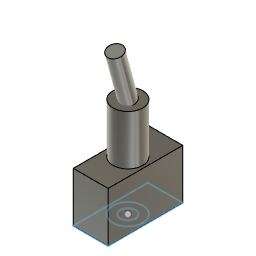
useless_box (Autodesk Fusion 360 archive; units mm, degrees)
design "small_switch"
Autodesk Fusion 360 part; units mm, degrees
note: some values were not read from the file. Chosen so that the rebuilt part matches the saved one: which bodies a step acts on; which face or edge a step refers to. Set by a fixed rule: which sketch regions a step uses.
sketch "Sketch1" plane through (0, 0, 0) normal (0, 0, 1) x (1, 0, 0)
  circle A0 centre (0, 0) radius 1.5
  circle A1 centre (0, 0) radius 3
  line L0 (3.5227, -7.5) -> (-3.4773, -7.5)
  line L1 (-3.4773, -7.5) -> (-3.4773, 7.5)
  line L2 (3.5227, 7.5) -> (3.5227, -7.5)
  line L3 (-3.4773, 7.5) -> (3.5227, 7.5)
  dimension "d20" = 6
  dimension "d29" = 3
  constraint horizontal L3
  constraint vertical L2
  constraint horizontal L0
  constraint vertical L1
  constraint concentric A0 A1
  measures "d20" diameter of A1
  measures "d29" diameter of A0
extrude "Extrude1" add sketch "Sketch1" along normal blind 30 and the other way blind -20 contours A0 makes body 1
extrude "Extrude2" add sketch "Sketch1" along normal blind 20 separate body contours A0 | A1 makes body 2
extrude "Extrude3" add sketch "Sketch1" along normal blind 10 separate body contours L0 L1 L2 L3 makes body 3
move_body "Move1" bodies 1 to x (1, 0, 0) y (0, 0.965926, 0.258819) z (0, -0.258819, 0.965926) at (0, 5.1764, 0.6815)

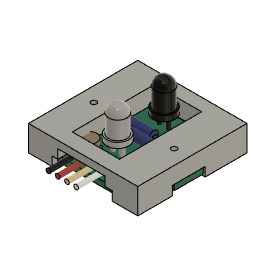
design "sensor"
Autodesk Fusion 360 part; units mm, degrees
sketch "Sketch1" plane through (0, 0, 0) normal (0, 0, 1) x (1, 0, 0)
  line L0 (0, 0) -> (15.24, 0)
  line L1 (15.24, 0) -> (15.24, 25.4)
  line L2 (15.24, 25.4) -> (0, 25.4)
  line L3 (0, 25.4) -> (0, 0)
  line L4 (2.54, 1.27) -> (12.7, 1.27)
  line L5 (12.7, 1.27) -> (12.7, 3.81)
  line L6 (12.7, 3.81) -> (2.54, 3.81)
  line L7 (2.54, 3.81) -> (2.54, 1.27)
  circle A0 centre (3.8195, 2.54) radius 0.635
  circle A1 centre (6.3595, 2.54) radius 0.635
  circle A2 centre (8.8995, 2.54) radius 0.635
  circle A3 centre (11.4395, 2.54) radius 0.635
  circle A4 centre (7.62, 8.89) radius 2.5
  line L8 (16.51, 21.59) -> (-7.62, 21.59) construction
  circle A5 centre (7.62, 21.59) radius 2.5
  line L9 (3.322, 17.78) -> (9.4206, 17.78)
  line L10 (9.4206, 17.78) -> (9.4206, 15.2896)
  line L11 (9.4206, 15.2896) -> (3.322, 15.2896)
  line L12 (3.322, 15.2896) -> (3.322, 17.78)
  circle A6 centre (6.35, 21.59) radius 0.635
  circle A7 centre (8.89, 21.59) radius 0.635
  circle A8 centre (6.35, 8.89) radius 0.635
  circle A9 centre (8.89, 8.89) radius 0.635
  circle A10 centre (6.35, 8.89) radius 0.635
  line L13 (11.8862, 12.7) -> (5.8127, 12.7)
  line L14 (5.8127, 12.7) -> (5.8127, 15.1867)
  line L15 (5.8127, 15.1867) -> (11.8862, 15.1867)
  line L16 (11.8862, 15.1867) -> (11.8862, 12.7)
  circle A11 centre (2.54, 16.51) radius 0.635
  circle A12 centre (10.16, 16.51) radius 0.635
  circle A13 centre (5.08, 13.97) radius 0.635
  circle A14 centre (12.7, 13.97) radius 0.635
  circle A15 centre (7.62, 8.89) radius 3
  circle A16 centre (7.62, 21.59) radius 3
  circle A17 centre (3.8195, 5.08) radius 0.635
  circle A18 centre (3.8195, 7.62) radius 0.635
  circle A19 centre (2.2166, 6.3624) radius 2.1559
  line L17 (-7, 17) -> (-7, 9)
  line L18 (-7, 17) -> (0, 17)
  line L19 (-7, 9) -> (0, 9)
  line L20 (15.24, 17) -> (23, 17)
  line L21 (23, 17) -> (23, 10)
  line L22 (23, 10) -> (23, 9)
  line L23 (23, 9) -> (15.24, 9)
  circle A20 centre (-3, 12.9629) radius 1.25
  circle A21 centre (19, 13) radius 1.25
  dimension "d1" = 15.24
  dimension "d2" = 25.4
  dimension "d3" = 1.27
  dimension "d6" = 7.62
  dimension "d7" = 0
  dimension "d8" = 5
  dimension "d9" = 5
  dimension "d10" = 1.27
  dimension "d11" = 1.27
  dimension "d12" = 1.27
  dimension "d13" = 1.27
  dimension "d14" = 1.27
  dimension "d15" = 1.27
  dimension "d16" = 1.27
  dimension "d17" = 1.27
  dimension "d18" = 1.27
  dimension "d19" = 6
  dimension "d20" = 6
  dimension "d43" = 1.27
  dimension "d44" = 1.27
  dimension "d53" = 2.5
  dimension "d54" = 2.5
  dimension "d55" = 22
  constraint horizontal L0
  constraint vertical L1
  constraint horizontal L2
  constraint vertical L3
  constraint coincident L0.start L3.end
  constraint horizontal L4
  constraint vertical L5
  constraint horizontal L6
  constraint vertical L7
  constraint perpendicular L1 L8
  constraint coincident L8 A5.centre
  constraint horizontal L9
  constraint vertical L10
  constraint horizontal L11
  constraint vertical L12
  constraint coincident L8 A6.centre
  constraint horizontal L13
  constraint vertical L14
  constraint horizontal L15
  constraint vertical L16
  constraint concentric A4 A15
  constraint concentric A5 A16
  constraint perpendicular L8 L17
  constraint coincident L3 L18.end
  constraint perpendicular L3 L18
  constraint coincident L3 L19.end
  constraint perpendicular L3 L19
  constraint coincident L1 L20.start
  constraint perpendicular L1 L20
  constraint perpendicular L20 L21
  constraint perpendicular L20 L22
  constraint coincident L1 L23.end
  constraint perpendicular L1 L23
  measures "d1" distance of L0.start L0.end
  measures "d2" distance of L0.start L2.end
  measures "d3" diameter of A0
  measures "d8" diameter of A4
  measures "d9" diameter of A5
  measures "d10" diameter of A6
  measures "d11" diameter of A7
  measures "d12" diameter of A8
  measures "d13" diameter of A9
  measures "d14" diameter of A10
  measures "d15" diameter of A11
  measures "d16" diameter of A12
  measures "d17" diameter of A13
  measures "d18" diameter of A14
  measures "d19" diameter of A15
  measures "d20" diameter of A16
  measures "d43" diameter of A17
  measures "d44" diameter of A18
  measures "d53" diameter of A20
  measures "d54" diameter of A21
  measures "d55" horizontal distance of A20.centre A21.centre
sketch "Sketch2" plane through (0, 0, 0) normal (1, 0, 0) x (0, 1, 0)
  arc A0 through (2.54, 0, 3.81) (2.168, 0.898, 3.81) (1.27, 1.27, 3.81)
  line L0 (-6.35, 1.27, 3.81) -> (1.27, 1.27, 3.81)
  arc A1 through (2.54, 0, 6.35) (2.168, 0.898, 6.35) (1.27, 1.27, 6.35)
  line L1 (-6.35, 1.27, 6.35) -> (1.27, 1.27, 6.35)
  arc A2 through (2.54, 0, 8.89) (2.168, 0.898, 8.89) (1.27, 1.27, 8.89)
  line L2 (-6.35, 1.27, 8.89) -> (1.27, 1.27, 8.89)
  arc A3 through (2.54, 0, 11.43) (2.168, 0.898, 11.43) (1.27, 1.27, 11.43)
  line L3 (-6.35, 1.27, 11.43) -> (1.27, 1.27, 11.43)
  circle A4 centre (16.51, 1.27) radius 1.25
  circle A5 centre (13.97, 1.27) radius 1.25
  dimension "d26" = 2.5
  dimension "d27" = 2.5
  measures "d26" diameter of A4
  measures "d27" diameter of A5
extrude "Extrude1" add sketch "Sketch1" along normal blind 6.5 contours A4 | A5 | A6 | A7 | A8 A10 | A9 makes body 1 at (10.1076, 21.3411, 4.3333) makes body 2 at (10.1076, 8.6411, 4.3333)
sphere "SpherePrimitive1" add diameter 5 placed x (-1, 0, 0) y (0, -1, 0) z (0, 0, 1) at (7.62, 21.59, 6.5) bodies 1
extrude "Extrude2" add sketch "Sketch1" along normal blind 1.5 contours A15 | A16 bodies 1 2
sphere "SpherePrimitive2" add diameter 5.0038 placed x (-1, 0, 0) y (0, -1, 0) z (0, 0, 1) at (7.62, 8.89, 6.5) bodies 2
sweep "Sweep1" add profiles "Sketch1" path "Sketch2" along L0 A0 section 1 contours A0 | A1 | A2 | A3 separate body makes body 3 at (6.9914, -1.27, 1.3332) makes body 4 at (9.5314, -1.27, 1.3332) makes body 5 at (4.4514, -1.27, 1.3332) makes body 6 at (12.0714, -1.27, 1.3332)
extrude "Extrude3" add sketch "Sketch2" along normal blind 9.906 and the other way blind -2.794 separate body contours A4 makes body 7
extrude "Extrude4" add sketch "Sketch2" along normal blind 12.446 and the other way blind -5.334 separate body contours A5 makes body 8
extrude "Extrude5" add sketch "Sketch1" along normal blind 2 separate body contours A17 A19 | A17 A18 A19 | A18 A19 picked at (3.5895, 4.9795) picked at (3.8746, 7.3788) makes body 9
extrude "Extrude6" add sketch "Sketch1" against normal blind 2.5 contours A0 | A1 | A2 | A3 | A6 | A7 | A8 A10 | A9 | A11 | A12 | A13 | A14 | A17 A19 | A17 A19 | A18 A19 | A18 A19 bodies 1 2 3 4 5 6 9 makes body 10 at (13.2418, 14.3011, -1.6667) makes body 11 at (4.5382, 13.6389, -1.6667) makes body 12 at (9.6736, 16.9182, -1.6667) makes body 13 at (1.9082, 16.4468, -1.6667)
extrude "Extrude7" add sketch "Sketch1" along normal blind 1.27 contours A11 | A12 | A13 | A14 bodies 7 8 10 11 12 13
extrude "Extrude8" add sketch "Sketch1" against normal blind 1.5 separate body contours L0 L1 L2 L3 | L3 L17 L18 L19 | L1 L20 L21 L22 L23 | L4 L5 L6 L7 | A0 | A1 | A2 | A3 | A4 | A5 | L9 L10 L11 L12 | A6 | A7 | A8 A10 | A9 | L13 L14 L15 L16 | A11 | A12 | A13 | A14 | A15 | A16 | A17 A19 | A17 A19 | A17 A18 A19 | A18 A19 | A18 A19 makes body 14
move_body "Move1" bodies 1 2 to x (1, 0, 0) y (0, 1, 0) z (0, 0, 1) at (0, 0, 3)
extrude "Extrude9" add 4 faces at (6.2674, 22.0322, 0.5) (9.0452, 21.8588, 0.5) (8.758, 8.5408, 0.5) (6.5249, 9.0092, 0.5) along direction (0, 0, -1) blind 3 on bodies 1 2 bodies 1 2
ref_plane "WorkPlane1" through (0, 0, 4.5) normal (0, 0, 1) x (1, 0, 0) in component "sensor_mount"
ref_plane "WorkPlane2" through (0, 0, 9.125) normal (0, 0, 1) x (1, 0, 0) in component "sensor_mount"
sketch "Sketch1 (2)" plane through (0, 0, 4.5) normal (0, 0, 1) x (1, 0, 0) in component "sensor_mount"
  line L0 (-7, 29) -> (23, 29)
  line L1 (23, 29) -> (23, -1)
  line L2 (23, -1) -> (-7, -1)
  line L3 (-7, -1) -> (-7, 29)
  line L4 (14, 32) -> (14, -1)
  line L5 (1.0449, -1) -> (1.0449, 29)
  line L6 (14, 25.5493) -> (1.0449, 25.5493)
  line L7 (14, 3) -> (1.0449, 3)
  circle A0 centre (19, 13) radius 0.75
  circle A1 centre (-3, 12.9629) radius 0.75
  line L8 (-0.5, 17.5) -> (-7, 17.5)
  line L9 (-0.5, 8.5) -> (-7, 8.5)
  line L10 (16, 8.5) -> (23, 8.5)
  line L11 (16, 17.5) -> (23, 17.5)
  line L12 (16, 17.5) -> (16, 29)
  line L13 (16, 8.5) -> (16, -1)
  line L14 (-0.5, 8.5) -> (-0.5, -1)
  line L15 (-0.5, 17.5) -> (-0.5, 29)
  point P0 (19, 13)
  point P1 (-3, 12.9629)
  dimension "d72" = 1.5
  dimension "d73" = 1.5
  constraint horizontal L0
  constraint vertical L1
  constraint horizontal L2
  constraint vertical L3
  constraint coincident L2 L4.end
  constraint perpendicular L2 L4
  constraint coincident L2 L5.start
  constraint coincident L0 L5.end
  constraint perpendicular L0 L5
  constraint coincident L4 L6.start
  constraint coincident L5 L6.end
  constraint perpendicular L5 L6
  constraint coincident L5 L7.end
  constraint perpendicular L5 L7
  constraint coincident P0 A0.centre
  constraint coincident P1 A1.centre
  constraint coincident L3 L8.end
  constraint perpendicular L3 L8
  constraint coincident L3 L9.end
  constraint perpendicular L3 L9
  constraint coincident L1 L10.end
  constraint perpendicular L1 L10
  constraint coincident L1 L11.end
  constraint perpendicular L1 L11
  constraint coincident L0 L12.end
  constraint perpendicular L0 L12
  constraint coincident L2 L13.end
  constraint perpendicular L2 L13
  constraint coincident L2 L14.end
  constraint perpendicular L2 L14
  constraint coincident L0 L15.end
  constraint perpendicular L0 L15
  measures "d72" diameter of A0
  measures "d73" diameter of A1
extrude "Extrude4'" add sketch "Sketch1 (2)" against normal blind 4.5 separate body contours L0 L3 L8 L15 | L0 L2 L3 L5 L8 L9 L14 L15 | L0 L4 L5 L6 | L2 L3 L9 L14 | L0 L1 L2 L4 L10 L11 L12 L13 | L0 L1 L11 L12 | L1 L2 L10 L13 makes body 15 in component "sensor_mount"
extrude "Extrude5'" add sketch "Sketch1 (2)" against normal blind 2 contours L2 L4 L5 L7 bodies 15 in component "sensor_mount"
extrude "Extrude6'" add sketch "Sketch1 (2)" against normal blind 7 contours L0 L3 L8 L15 | L2 L3 L9 L14 | L0 L1 L11 L12 | L1 L2 L10 L13 bodies 15 in component "sensor_mount"
component "sensor_mount" placed x (1, 0, 0) y (0, 1, 0) z (0, 0, 1) at (0, 0, 0)
named bodies: "detector", "emitter", "wire2", "wire3", "wire1", "wir45", "res1", "res2", "cap", "board"

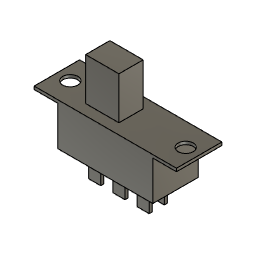
design "slide_switch"
Autodesk Fusion 360 part; units mm, degrees
sketch "Sketch1" plane through (0, 0, 0) normal (0, 0, 1) x (1, 0, 0)
  line L0 (11.75, 3.75) -> (-11.75, 3.75)
  line L1 (-11.75, 3.75) -> (-11.75, -3.75)
  line L2 (-11.75, -3.75) -> (11.75, -3.75)
  line L3 (11.75, -3.75) -> (11.75, 3.75)
  line L4 (11.75, 3.75) -> (-11.75, -3.75) construction
  line L5 (-11.75, 3.75) -> (11.75, -3.75) construction
  line L6 (7.85, -3.75) -> (-7.85, -3.75)
  line L7 (-7.85, -3.75) -> (-7.85, 3.75)
  line L8 (-7.85, 3.75) -> (7.85, 3.75)
  line L9 (7.85, 3.75) -> (7.85, -3.75)
  line L10 (7.85, -3.75) -> (-7.85, 3.75) construction
  line L11 (-7.85, -3.75) -> (7.85, 3.75) construction
  line L12 (9.525, -3.75) -> (-9.525, -3.75) construction
  line L13 (-9.525, -3.75) -> (-9.525, 3.75) construction
  line L14 (-9.525, 3.75) -> (9.525, 3.75) construction
  line L15 (9.525, 3.75) -> (9.525, -3.75) construction
  line L16 (9.525, -3.75) -> (-9.525, 3.75) construction
  line L17 (-9.525, -3.75) -> (9.525, 3.75) construction
  circle A0 centre (-9.525, 0) radius 1.25
  circle A1 centre (9.525, 0) radius 1.25
  line L18 (5, 2) -> (-5, 2) construction
  line L19 (-5, 2) -> (-5, -2) construction
  line L20 (-5, -2) -> (5, -2) construction
  line L21 (5, -2) -> (5, 2) construction
  line L22 (5, 2) -> (-5, -2) construction
  line L23 (-5, 2) -> (5, -2) construction
  line L24 (-5, 2) -> (0.5, 2)
  line L25 (0.5, 2) -> (0.5, -2)
  line L26 (0.5, -2) -> (-5, -2)
  line L27 (-5, -2) -> (-5, 2)
  dimension "d1" = 23.5
  dimension "d2" = 7.5
  dimension "d3" = 15.7
  dimension "d4" = 19.05
  dimension "d5" = 2.5
  dimension "d6" = 2.5
  dimension "d7" = 10
  dimension "d8" = 4
  dimension "d9" = 5.5
  constraint horizontal L0
  constraint perpendicular L0 L1
  constraint parallel L0 L2
  constraint parallel L1 L3
  constraint coincident L4 origin
  constraint coincident L5 origin
  constraint horizontal L6
  constraint perpendicular L6 L7
  constraint parallel L6 L8
  constraint parallel L7 L9
  constraint coincident L10 origin
  constraint coincident L11 origin
  constraint coincident L2 L6.start
  constraint horizontal L12
  constraint perpendicular L12 L13
  constraint parallel L12 L14
  constraint parallel L13 L15
  constraint coincident L16 origin
  constraint coincident L17 origin
  constraint midpoint L13 A0.centre
  constraint midpoint L15 A1.centre
  constraint horizontal L18
  constraint perpendicular L18 L19
  constraint parallel L18 L20
  constraint parallel L19 L21
  constraint coincident L22 origin
  constraint coincident L23 origin
  constraint horizontal L24
  constraint vertical L25
  constraint horizontal L26
  constraint vertical L27
  measures "d1" distance of L1.end L2.end
  measures "d2" distance of L0.end L1.end
  measures "d3" distance of L7.end L8.end
  measures "d4" distance of L13.end L14.end
  measures "d5" diameter of A0
  measures "d6" diameter of A1
  measures "d7" distance of L19.end L20.end
  measures "d8" distance of L18.end L19.end
  measures "d9" distance of L18.end L24.end
extrude "Extrude1" add sketch "Sketch1" against normal blind 7 contours L0 L2 L6 L7 L8 L9 | L24 L25 L26 L27 makes body 1
extrude "Extrude2" add sketch "Sketch1" against normal blind 0.5 contours L0 L2 L3 L9 | L0 L1 L2 L7 bodies 1
extrude "Extrude3" add sketch "Sketch1" along normal blind 7 separate body contours L24 L25 L26 L27 makes body 2
sketch "Sketch2" plane through (0, 0, -7) normal (0, 0, -1) x (1, 0, 0)
  line L0 (-7.85, -3.75) -> (7.85, -3.75)
  line L1 (7.85, -3.75) -> (7.85, 3.75)
  line L2 (7.85, 3.75) -> (-7.85, 3.75)
  line L3 (-7.85, 3.75) -> (-7.85, -3.75)
  line L4 (-5, 1.5) -> (5, 1.5) construction
  line L5 (5, 1.5) -> (5, -1.5) construction
  line L6 (5, -1.5) -> (-5, -1.5) construction
  line L7 (-5, -1.5) -> (-5, 1.5) construction
  line L8 (-5, 1.5) -> (5, -1.5) construction
  line L9 (5, 1.5) -> (-5, -1.5) construction
  line L10 (-5, 1.5) -> (-3, 1.5)
  line L11 (-3, 1.5) -> (-3, 1)
  line L12 (-3, 1) -> (-5, 1)
  line L13 (-5, 1) -> (-5, 1.5)
  line L14 (-5, -1) -> (-3, -1)
  line L15 (-3, -1) -> (-3, -1.5)
  line L16 (-3, -1.5) -> (-5, -1.5)
  line L17 (-5, -1.5) -> (-5, -1)
  line L18 (-5, 1) -> (-5, 1.5)
  line L19 (-5, 1.5) -> (-3, 1.5)
  line L20 (-3, 1.5) -> (-3, 1)
  line L21 (-3, 1) -> (-5, 1)
  line L22 (5, 1.5) -> (-5, -1.5) construction
  line L23 (3, 1.5) -> (5, 1.5)
  line L24 (5, 1.5) -> (5, 1)
  line L25 (5, 1) -> (3, 1)
  line L26 (3, 1) -> (3, 1.5)
  line L27 (5, -1.5) -> (3, -1.5)
  line L28 (3, -1.5) -> (3, -1)
  line L29 (5, -1) -> (5, -1.5)
  line L30 (3, -1) -> (5, -1)
  line L31 (-1, 1.5) -> (1, 1.5)
  line L32 (1, 1.5) -> (1, 1)
  line L33 (1, 1) -> (-1, 1)
  line L34 (-1, 1) -> (-1, 1.5)
  line L35 (1, -1.5) -> (-1, -1.5)
  line L36 (-1, -1.5) -> (-1, -1)
  line L37 (1, -1) -> (1, -1.5)
  line L38 (-1, -1) -> (1, -1)
  dimension "d16" = 10
  dimension "d17" = 3
  dimension "d18" = 2
  dimension "d19" = 0.5
  dimension "d20" = 2
  dimension "d21" = 0.5
  dimension "d22" = 2
  dimension "d23" = 0.5
  dimension "d24" = 2
  dimension "d25" = 0.5
  dimension "d26" = 2
  dimension "d27" = 0.5
  dimension "d28" = 2
  dimension "d29" = 0.5
  dimension "d30" = 2
  dimension "d31" = 0.5
  constraint horizontal L4
  constraint perpendicular L4 L5
  constraint parallel L4 L6
  constraint parallel L5 L7
  constraint coincident L8 origin
  constraint coincident L9 origin
  constraint horizontal L10
  constraint vertical L11
  constraint horizontal L12
  constraint vertical L13
  constraint horizontal L14
  constraint vertical L15
  constraint horizontal L16
  constraint vertical L17
  constraint horizontal L19
  constraint vertical L20
  constraint horizontal L21
  constraint vertical L18
  constraint horizontal L23
  constraint vertical L24
  constraint horizontal L25
  constraint vertical L26
  constraint horizontal L30
  constraint vertical L29
  constraint horizontal L27
  constraint vertical L28
  constraint horizontal L31
  constraint vertical L32
  constraint horizontal L33
  constraint vertical L34
  constraint horizontal L38
  constraint vertical L37
  constraint horizontal L35
  constraint vertical L36
  measures "d16" distance of L5.end L6.end
  measures "d17" distance of L4.end L5.end
  measures "d18" distance of L4.start L10.end
  measures "d19" distance of L4.start L12.end
  measures "d20" distance of L14.end L14.start
  measures "d21" distance of L6.end L14.start
  measures "d22" distance of L10.end L4.start
  measures "d23" distance of L12.end L4.start
  measures "d24" distance of L4.end L23.start
  measures "d25" distance of L25.end L23.start
  measures "d26" distance of L28.end L29.start
  measures "d27" distance of L27.end L28.end
  measures "d28" distance of L31.end L31.start
  measures "d29" distance of L33.end L31.start
  measures "d30" distance of L36.end L37.start
  measures "d31" distance of L35.end L36.end
extrude "Extrude4" add sketch "Sketch2" along normal blind 4 contours L10 L11 L12 L13 L18 L19 L20 L21 | L14 L15 L16 L17 | L23 L24 L25 L26 | L27 L28 L29 L30 | L31 L32 L33 L34 | L35 L36 L37 L38 bodies 1 2
copy_body "Body->Comp1" bodies 1 removing the originals makes body 4 in component "body"
copy_body "Body->Comp2" bodies 2 removing the originals makes body 5 in component "slider"
component "body" placed x (1, 0, 0) y (0, 1, 0) z (0, 0, 1) at (0, 0, 0)
component "slider" placed x (1, 0, 0) y (0, 1, 0) z (0, 0, 1) at (0, 0, 0)
named bodies: "body", "slider"

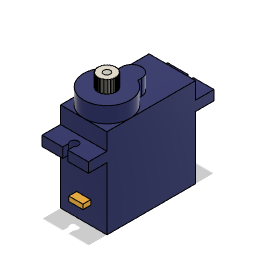
design "blue_SG90"
Autodesk Fusion 360 part; units mm, degrees
sketch "Left" plane through (0, 0, 0) normal (1, 0, 0) x (0, 0, -1)
  line L0 (-21.4055, -22.0984) -> (1.0945, -22.0984)
  line L1 (-21.4055, 4.6016) -> (1.0945, 4.6016)
  line L2 (-21.4055, 0.6016) -> (1.0945, 0.6016)
  line L3 (-21.4055, 0.6016) -> (-21.4055, 4.6016)
  line L4 (5.7945, -22.0984) -> (5.7945, -6.1984)
  line L5 (-26.1055, -6.1984) -> (-26.1055, -3.6984)
  line L6 (-26.1055, -3.6984) -> (-21.4055, -3.6984)
  line L7 (1.0945, -3.6984) -> (5.7945, -3.6984)
  line L8 (-26.1055, -6.1984) -> (-21.4055, -6.1984)
  line L9 (1.0945, -6.1984) -> (5.7945, -6.1984)
  line L10 (1.0945, -22.0984) -> (1.0945, -6.1984)
  line L11 (1.0945, -3.6984) -> (1.0945, 0.6016)
  line L12 (-21.4055, -22.0984) -> (-21.4055, -6.1984)
  line L13 (-21.4055, -3.6984) -> (-21.4055, 0.6016)
  line L14 (-15.5055, 0.6016) -> (-15.5055, 13)
  line L15 (-6.7055, 0.6016) -> (-6.7055, 13)
  line L16 (1.0945, -22.0984) -> (1.0945, -6.1984)
  line L17 (1.0945, -3.6984) -> (1.0945, 13)
  line L18 (5.7945, -3.6984) -> (5.7945, -6.1984)
  dimension "d1" = 22.5
  dimension "d2" = 26.7
  dimension "d3" = 22.7
  dimension "d4" = 4
  dimension "d5" = 22.7
  dimension "d13" = 5.9
  constraint perpendicular L1 L3
  constraint parallel L0 L6
  constraint parallel L0 L8
  constraint parallel L5 L12
  constraint coincident L6.end L12
  constraint coincident L7.start L10
  constraint collinear L6 L7
  constraint collinear L8 L9
  constraint parallel L4 L10
  constraint collinear L10 L11
  constraint collinear L12 L13
  constraint parallel L3 L14
  constraint parallel L14 L16
  constraint collinear L16 L17
  constraint parallel L14 L15
  constraint coincident L2 L15.start
  constraint coincident L2 L14.start
  constraint perpendicular L9 L18
  measures "d1" distance of L0.start L0.end
  measures "d4" distance of L1.start L2.start
  measures "d5" distance of L0.start L2.start
  measures "d13" distance of L3 L14
extrude "Extrude1" add sketch "Left" along normal mid plane 11.8 contours L0 L2 L5 L6 L7 L8 L9 L10 L11 L12 L13 L16 L17 L18 makes body 1
sketch "TOP" plane through (0, 0.6016, 0) normal (0, 1, 0) x (-1, 0, 0)
  line L0 (5.9, 21.4055) -> (-5.9, 21.4055)
  line L1 (-5.9, 21.4055) -> (-5.9, -1.0945)
  line L2 (-5.9, -1.0945) -> (5.9, -1.0945)
  line L3 (5.9, -1.0945) -> (5.9, 21.4055)
  circle A0 centre (0, 15.5055) radius 2.3
  circle A1 centre (0, 15.5055) radius 0.85
  line L4 (0, -1.0945) -> (0, 27)
  line L5 (0, 27) -> (0, -1.0945)
  arc A2 (-2.5, 9.2055) -> (2.5, 9.2055) centre (0, 9.2055) ccw
  line L6 (-2.5, 9.2055) -> (-2.5, 10.1613)
  line L7 (2.5, 9.2055) -> (2.5, 10.1613)
  arc A3 (2.5, 10.1613) -> (-2.5, 10.1613) centre (0, 15.5055) ccw
  line L8 (5.9, -5.7945) -> (-5.9, -5.7945)
  line L9 (-0.65, -4.2545) -> (-0.65, -5.7945)
  line L10 (0.65, -4.2545) -> (0.65, -5.7945)
  arc A4 (0.65, -4.2545) -> (-0.65, -4.2545) centre (0, -3.4945) ccw
  line L11 (5.9, 26.1055) -> (-5.9, 26.1055)
  arc A5 (-0.65, 24.5654) -> (0.65, 24.5654) centre (0, 23.8055) ccw
  line L12 (0.65, 24.5654) -> (0.65, 26.1055)
  line L13 (-0.65, 24.5654) -> (-0.65, 26.1055)
  point P0 (0, 15.5055)
  point P1 (0, 6.7055)
  point P2 (0, -1.0945)
  point P3 (5.9, -5.7945)
  point P4 (-5.9, -5.7945)
  point P5 (0, -5.7945)
  point P6 (5.9, 26.1055)
  point P7 (-5.9, 26.1055)
  point P8 (0, 26.1055)
  point P9 (0, 21.4055)
  dimension "d16" = 4.6
  dimension "d17" = 1.7
  dimension "d18" = 11.8
  dimension "d27" = 2
  dimension "d31" = 2
  constraint coincident P0 A0.centre
  constraint concentric A1 A3
  constraint coincident P1 A2
  constraint coincident P2 L4.start
  constraint perpendicular L0 L4
  constraint parallel L4 L6
  constraint parallel L4 L7
  constraint coincident P3 L8.start
  constraint coincident P4 L8.end
  constraint coincident P6 L11.start
  constraint coincident P7 L11.end
  constraint coincident L11 L12.end
  constraint coincident L11 L13.end
  measures "d16" diameter of A0
  measures "d17" diameter of A1
  measures "d18" diameter of A3
  measures "d27" diameter of A4
  measures "d31" diameter of A5
extrude "Extrude2" add sketch "TOP" along normal blind 4 contours A0 L4 L5 A2 L7 A3 | A0 L4 L5 A2 L6 A3 bodies 1
extrude "Extrude3" add sketch "TOP" along normal blind 7.2 separate body contours A0 A1 L4 L5 | A0 A1 L4 L5 makes body 2
extrude "Extrude4" cut sketch "TOP" against normal through all contours L4 L5 L11 A5 L13 | L4 L5 L11 A5 L12 bodies 1
extrude "Extrude5" cut sketch "TOP" against normal through all contours L8 L9 L10 A4 bodies 1
sketch "Front" plane through (0, 0, 21.4055) normal (0, 0, 1) x (1, 0, 0)
  line L0 (-5.9, -22.0984) -> (5.9, -22.0984)
  line L1 (5.9, -22.0984) -> (5.9, -6.1984)
  line L2 (5.9, -6.1984) -> (-5.9, -6.1984)
  line L3 (-5.9, -6.1984) -> (-5.9, -22.0984)
  line L4 (-1.8, -17.5984) -> (1.8, -17.5984)
  line L5 (0, -22.0984) -> (0, -6.1984)
  line L6 (1.8, -17.5984) -> (1.8, -16.3984)
  line L7 (-1.8, -17.5984) -> (-1.8, -16.3984)
  line L8 (-1.8, -16.3984) -> (1.8, -16.3984)
extrude "Extrude6" add sketch "Front" along normal blind 2 separate body contours L4 L5 L6 L8 | L4 L5 L7 L8 makes body 3
copy_body "Body->Comp1" bodies 3 removing the originals makes body 4 in component "connector"
copy_body "Body->Comp2" bodies 2 removing the originals makes body 5 in component "shaft"
copy_body "Body->Comp3" bodies 1 removing the originals makes body 6 in component "body\\"
sketch "Sketch1" plane through (0, 7.8016, 0) normal (0, 1, 0) x (-1, 0, 0) in component "shaft"
  circle A0 centre (0, 15.5055) radius 0.85
  circle A1 centre (0, 15.5055) radius 2.3
  circle A2 centre (0, 15.5055) radius 2.3
  circle A3 centre (-0.0134, 13.2055) radius 0.125
  dimension "d42" = 0.25
  constraint coincident A2 A3.centre
  measures "d42" diameter of A3
extrude "Extrude1'" cut sketch "Sketch1" against normal up to surface (3.2 mm away) contours A1 A2 A3 | A1 A2 A3 picked at (-0.0101, 13.2473) picked at (-0.0141, 13.1641) bodies 5 in component "shaft"
pattern_circular "C-Pattern1" count 28 over 360 about axis through (0, 15.4797, 15.5055) along (0, -1, 0) of "Extrude1'" in component "shaft"
component "connector" placed x (1, 0, 0) y (0, 1, 0) z (0, 0, 1) at (0, 0, 0)
component "shaft" placed x (1, 0, 0) y (0, 1, 0) z (0, 0, 1) at (0, 0, 0)
component "body\\" placed x (1, 0, 0) y (0, 1, 0) z (0, 0, 1) at (0, 0, 0)

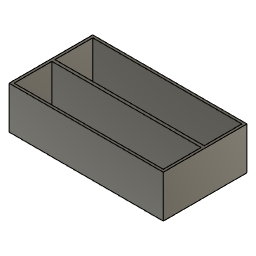
design "battery_holder"
Autodesk Fusion 360 part; units mm, degrees
sketch "Sketch1" plane through (0, 0, 0) normal (0, 0, 1) x (1, 0, 0)
  line L0 (38.25, 20.75) -> (-38.25, 20.75)
  line L1 (-38.25, 20.75) -> (-38.25, -20.75)
  line L2 (-38.25, -20.75) -> (38.25, -20.75)
  line L3 (38.25, -20.75) -> (38.25, 20.75)
  line L4 (38.25, 20.75) -> (-38.25, -20.75) construction
  line L5 (-38.25, 20.75) -> (38.25, -20.75) construction
  line L6 (-37, 19.5) -> (37, 19.5)
  line L7 (37, 19.5) -> (37, -19.5)
  line L8 (37, -19.5) -> (-37, -19.5)
  line L9 (-37, -19.5) -> (-37, 19.5)
  line L10 (-37, 19.5) -> (37, -19.5) construction
  line L11 (37, 19.5) -> (-37, -19.5) construction
  line L12 (37, -0.75) -> (-37, -0.75)
  line L13 (-37, -0.75) -> (-37, 0.75)
  line L14 (-37, 0.75) -> (37, 0.75)
  line L15 (37, 0.75) -> (37, -0.75)
  line L16 (37, -0.75) -> (-37, 0.75) construction
  line L17 (-37, -0.75) -> (37, 0.75) construction
  line L18 (0, 0) -> (0, 10) construction
  line L19 (0, 0) -> (0, -10) construction
  circle A0 centre (0, -10) radius 1.5
  circle A1 centre (0, 10) radius 1.5
  dimension "d1" = 76.5
  dimension "d2" = 41.5
  dimension "d3" = 74
  dimension "d4" = 39
  dimension "d5" = 1.5
  dimension "d10" = 10
  dimension "d11" = 10
  dimension "d12" = 3
  dimension "d13" = 3
  constraint horizontal L0
  constraint perpendicular L0 L1
  constraint parallel L0 L2
  constraint parallel L1 L3
  constraint coincident L4 L18.start
  constraint coincident L5 L18.start
  constraint coincident L18.start L19.start
  constraint horizontal L6
  constraint perpendicular L6 L7
  constraint parallel L6 L8
  constraint parallel L7 L9
  constraint coincident L10 L18.start
  constraint coincident L11 L18.start
  constraint horizontal L12
  constraint perpendicular L12 L13
  constraint parallel L12 L14
  constraint parallel L13 L15
  constraint coincident L16 L18.start
  constraint coincident L17 L18.start
  constraint vertical L18
  constraint vertical L19
  constraint coincident L19.end A0.centre
  constraint coincident L18.end A1.centre
  measures "d1" distance of L1.end L2.end
  measures "d2" distance of L0.end L1.end
  measures "d3" distance of L7.end L8.end
  measures "d4" distance of L6.end L7.end
  measures "d5" distance of L12.end L13.end
  measures "d10" distance of L18.start L18.end
  measures "d11" distance of L18.start L19.end
  measures "d12" diameter of A0
  measures "d13" diameter of A1
extrude "Extrude1" add sketch "Sketch1" along normal blind 21 contours L0 L1 L2 L3 | L7 L9 L12 L13 L14 L15
extrude "Extrude2" add sketch "Sketch1" along normal blind 1.5 contours L6 L7 L9 L14 | L7 L8 L9 L12

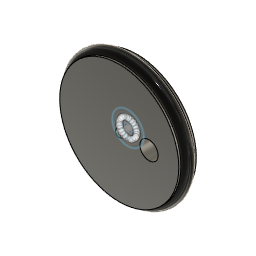
design "wheel"
Autodesk Fusion 360 part; units mm, degrees
sketch "servo splines" plane through (0, 0, 0) normal (0, 1, 0) x (1, 0, 0)
  circle A0 centre (0, 0) radius 1.1
  circle A1 centre (0, 0) radius 4.5
  circle A2 centre (0, 0) radius 2.2
  line L0 (-0.9545, -1.9821) -> (-0.822, -2.361)
  line L1 (1.72, 1.3717) -> (2.1189, 1.3267)
  line L2 (0.9545, -1.9821) -> (0.822, -2.361)
  line L3 (2.1448, -0.4895) -> (2.3584, -0.8294)
  line L4 (-1.9053, -1.1) -> (-2.293, -0.9961)
  line L5 (-2.1448, -0.4895) -> (-2.4847, -0.276)
  line L6 (-1.4964, -1.6127) -> (-1.4814, -2.0138)
  line L7 (-0.3279, -2.1754) -> (-0.6509, -2.4138)
  line L8 (-2.0479, 0.8038) -> (-2.2084, 1.1717)
  line L9 (-1.2393, 1.8177) -> (-1.6337, 1.8924)
  line L10 (0.9545, -1.9821) -> (1.3334, -2.1147)
  line L11 (2.1938, 0.1644) -> (2.4557, 0.4687)
  line L12 (-1.9053, -1.1) -> (-2.0091, -1.4877)
  line L13 (1.9053, -1.1) -> (2.0091, -1.4877)
  line L14 (0.3279, -2.1754) -> (0.0895, -2.4984)
  line L15 (1.2393, 1.8177) -> (1.6337, 1.8924)
  line L16 (0.6485, 2.1023) -> (0.4609, 2.4571)
  line L17 (-2.1938, 0.1644) -> (-2.4981, -0.0974)
  line L18 (0, 2.2) -> (-0.2838, 2.4838)
  line L19 (-1.4964, -1.6127) -> (-1.8975, -1.6277)
  line L20 (-1.2393, 1.8177) -> (-1.1647, 2.2121)
  line L21 (-1.72, 1.3717) -> (-2.1189, 1.3267)
  line L22 (0, 2.2) -> (0.2838, 2.4838)
  line L23 (1.2393, 1.8177) -> (1.1647, 2.2121)
  line L24 (-1.72, 1.3717) -> (-1.765, 1.7706)
  line L25 (-0.6485, 2.1023) -> (-1.0033, 2.2898)
  line L26 (2.1448, -0.4895) -> (2.4847, -0.276)
  line L27 (0, 0) -> (0, 4.5) construction
  circle A3 centre (0, 0) radius 2.5
  line L28 (-0.3279, -2.1754) -> (-0.0895, -2.4984)
  line L29 (2.0479, 0.8038) -> (2.2084, 1.1717)
  line L30 (2.0479, 0.8038) -> (2.4158, 0.6432)
  line L31 (1.9053, -1.1) -> (2.293, -0.9961)
  line L32 (-2.1448, -0.4895) -> (-2.3584, -0.8294)
  line L33 (1.4964, -1.6127) -> (1.8975, -1.6277)
  line L34 (0.3279, -2.1754) -> (0.6509, -2.4138)
  line L35 (-0.9545, -1.9821) -> (-1.3334, -2.1147)
  line L36 (1.4964, -1.6127) -> (1.4814, -2.0138)
  line L37 (1.72, 1.3717) -> (1.765, 1.7706)
  line L38 (-2.0479, 0.8038) -> (-2.4158, 0.6432)
  line L39 (-0.6485, 2.1023) -> (-0.4609, 2.4571)
  line L40 (2.1938, 0.1644) -> (2.4981, -0.0974)
  line L41 (0.6485, 2.1023) -> (1.0033, 2.2898)
  line L42 (-2.1938, 0.1644) -> (-2.4557, 0.4687)
  dimension "d2" = 360
  dimension "d252_1" = 5
  dimension "d253_1" = 4.4
  dimension "d254_1" = 2.2
  dimension "d255_1" = 135
  dimension "d256_1" = 90
  constraint concentric A1 A3
  constraint concentric A1 A2
  constraint concentric A0 A1
  constraint coincident A0.centre A1.centre
  constraint coincident L27.end A1
  constraint vertical L27
  constraint coincident L18.start L27
  constraint coincident L18.start A2
  constraint coincident L18.end A3
  constraint coincident L22.end A3
  measures "d252_1" diameter of A3
  measures "d253_1" diameter of A2
  measures "d254_1" diameter of A0
  measures "d255_1" angle of L18 L27
  measures "d256_1" angle of L18 L22
sketch "wheel" plane through (0, 0, 0) normal (0, 1, 0) x (1, 0, 0)
  circle A0 centre (0, 0) radius 17
  line L0 (0, 0) -> (8.5, 0) construction
  circle A1 centre (8.5, 0) radius 2.6
  dimension "d8" = 34
  dimension "d29" = 8.5
  dimension "d30" = 5.2
  constraint coincident A0.centre L0.start
  constraint horizontal L0
  constraint coincident L0.end A1.centre
  measures "d8" diameter of A0
  measures "d29" distance of A0.centre L0.end
  measures "d30" diameter of A1
sketch "o_ring_profile" plane through (0, 0, 0) normal (1, 0, 0) x (0, 1, 0)
  line L0 (0, -17) -> (0, 17)
  circle A0 centre (0, 17) radius 1.5
  circle A1 centre (0, -17) radius 1.5 construction
  line L1 (0, -15) -> (1.9, -17)
  line L2 (1.9, -17) -> (2.5, -17)
  line L3 (2.5, -17) -> (2.5, -18.5)
  line L4 (2.5, -18.5) -> (-2.5, -18.5)
  line L5 (-2.5, -18.5) -> (-2.5, -17)
  line L6 (-2.5, -17) -> (-1.9, -17)
  line L7 (-1.9, -17) -> (0, -15)
  dimension "d9" = 3
  dimension "d18" = 3
  constraint coincident L0.end A0.centre
  constraint coincident L0.start A1.centre
  constraint coincident L0 L1.start
  constraint perpendicular L0 L2
  constraint perpendicular L2 L3
  constraint perpendicular L3 L4
  constraint perpendicular L4 L5
  constraint perpendicular L5 L6
  measures "d9" diameter of A0
  measures "d18" diameter of A1
extrude "Extrude1" add sketch "wheel" along normal mid plane 5 makes body 1
sweep "Sweep2" cut profiles "o_ring_profile" path "wheel" along A0 section 1 contours L1 L2 L3 L4 L5 L6 L7 bodies 1
extrude "Extrude2" cut sketch "servo splines" along normal blind 2.5 contours A0 | A2 | A2 L26 A3 L40 | A2 L11 A3 L30 | A2 L3 A3 L31 | A2 L1 A3 L29 | A2 L13 A3 L33 | A2 L15 A3 L37 | A2 L10 A3 L36 | A2 L23 A3 L41 | A2 L2 A3 L34 | A2 L16 L22 A3 | A2 L14 A3 L28 | A2 L18 A3 L39 | A2 L0 L7 A3 | A2 L20 L25 A3 | A2 L6 A3 L35 | A2 L9 L24 A3 | A2 L12 L19 A3 | A2 L8 L21 A3 | A2 L4 A3 L32 | A2 A3 L38 L42 | A2 L5 L17 A3 bodies 1
extrude "Extrude3" cut sketch "servo splines" against normal blind 2.5 contours A0 bodies 1
sweep "Sweep1" add profiles "o_ring_profile" path "wheel" along A0 section 1 contours A0 separate body makes body 2
named bodies: "o-ring", "wheel"
